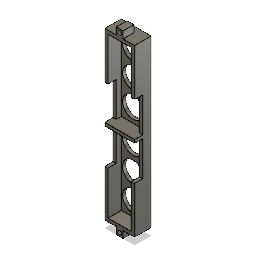
_Tamed Tiger.d4603d96-84c6-47e9-a002-08c8963379fb (Autodesk Fusion 360 design; units mm, degrees)
Autodesk Fusion 360 part; units mm, degrees
sketch "Sketch1" plane through (0, 0, 0) normal (0, 0, 1) x (1, 0, 0) in component "Chassis"
  line L0 (0, 0) -> (142, 0)
  line L1 (142, 0) -> (142, 170)
  line L2 (142, 170) -> (0, 170)
  line L3 (0, 170) -> (0, 0)
  line L4 (3, 3) -> (139, 3)
  line L5 (139, 3) -> (139, 167)
  line L6 (139, 167) -> (3, 167)
  line L7 (3, 167) -> (3, 3)
  line L8 (35, 154) -> (55, 154)
  line L9 (58, 86.5) -> (32, 86.5)
  line L10 (35, 86.5) -> (35, 142)
  line L11 (32, 142) -> (32, 167)
  line L12 (32, 157) -> (58, 157)
  line L13 (58, 167) -> (58, 85)
  line L14 (32, 85) -> (32, 142)
  line L15 (58, 3) -> (58, 85)
  line L16 (35, 83.5) -> (35, 28)
  line L17 (32, 28) -> (32, 3)
  line L18 (32, 13) -> (58, 13)
  line L19 (35, 16) -> (55, 16)
  line L20 (32, 85) -> (32, 28)
  line L21 (35, 142) -> (35, 154)
  line L22 (35, 157) -> (35, 167)
  line L23 (55, 167) -> (55, 157)
  line L24 (55, 154) -> (55, 86.5)
  line L25 (35, 28) -> (35, 16)
  line L26 (35, 13) -> (35, 3)
  line L27 (55, 3) -> (55, 13)
  line L28 (55, 16) -> (55, 83.5)
  line L29 (84, 86.5) -> (110, 86.5)
  line L30 (87, 154) -> (87, 86.5)
  line L31 (107, 86.5) -> (107, 142)
  line L32 (84, 167) -> (84, 85)
  line L33 (110, 28) -> (110, 3)
  line L34 (107, 157) -> (107, 167)
  line L35 (107, 16) -> (87, 16)
  line L36 (110, 85) -> (110, 142)
  line L37 (110, 157) -> (84, 157)
  line L38 (87, 167) -> (87, 157)
  line L39 (110, 13) -> (84, 13)
  line L40 (87, 3) -> (87, 13)
  line L41 (107, 28) -> (107, 16)
  line L42 (107, 142) -> (107, 154)
  line L43 (87, 16) -> (87, 83.5)
  line L44 (107, 83.5) -> (107, 28)
  line L45 (110, 85) -> (110, 28)
  line L46 (107, 154) -> (87, 154)
  line L47 (107, 13) -> (107, 3)
  line L48 (110, 142) -> (110, 167)
  line L49 (84, 3) -> (84, 85)
  line L50 (45, 163) -> (48, 163)
  line L51 (48, 163) -> (42, 163)
  line L52 (42, 163) -> (42, 157)
  line L53 (42, 157) -> (48, 157)
  line L54 (48, 157) -> (48, 163)
  line L55 (97, 163) -> (100, 163)
  line L56 (100, 163) -> (94, 163)
  line L57 (94, 163) -> (94, 157)
  line L58 (94, 157) -> (100, 157)
  line L59 (100, 157) -> (100, 163)
  line L60 (97, 7) -> (100, 7)
  line L61 (45, 7) -> (48, 7)
  line L62 (48, 7) -> (42, 7)
  line L63 (42, 7) -> (42, 13)
  line L64 (42, 13) -> (48, 13)
  line L65 (48, 13) -> (48, 7)
  line L66 (100, 7) -> (94, 7)
  line L67 (94, 7) -> (94, 13)
  line L68 (94, 13) -> (100, 13)
  line L69 (100, 13) -> (100, 7)
  line L70 (110, 83.5) -> (84, 83.5)
  line L71 (58, 83.5) -> (32, 83.5)
  line L72 (58, 53.5) -> (55, 53.5)
  line L73 (35, 53.5) -> (32, 53.5)
  line L74 (58, 116.5) -> (55, 116.5)
  line L75 (35, 116.5) -> (32, 116.5)
  line L76 (84, 116.5) -> (87, 116.5)
  line L77 (107, 116.5) -> (110, 116.5)
  line L78 (110, 53.5) -> (107, 53.5)
  line L79 (87, 53.5) -> (84, 53.5)
  line L80 (84, 3) -> (58, 3)
  line L81 (58, 3) -> (58, 6)
  line L82 (58, 6) -> (84, 6)
  line L83 (84, 6) -> (84, 3)
  line L84 (84, 167) -> (58, 167)
  line L85 (58, 167) -> (58, 164)
  line L86 (58, 164) -> (84, 164)
  line L87 (84, 164) -> (84, 167)
  line L88 (136, 80) -> (139, 80)
  line L89 (136, 90) -> (139, 90)
  line L90 (139, 90) -> (136, 90)
  line L91 (136, 90) -> (136, 80)
  line L92 (136, 80) -> (139, 80)
  line L93 (139, 80) -> (139, 90)
  line L94 (6, 85) -> (6, 90)
  line L95 (6, 90) -> (3, 90)
  line L96 (3, 90) -> (3, 80)
  line L97 (3, 80) -> (6, 80)
  line L98 (6, 80) -> (6, 90)
  line L99 (84, 90) -> (81, 90)
  line L100 (81, 90) -> (84, 90)
  line L101 (81, 80) -> (84, 80)
  line L102 (81, 80) -> (84, 80)
  line L103 (84, 80) -> (84, 90)
  line L104 (58, 90) -> (58, 80)
  line L105 (58, 80) -> (61, 80)
  line L106 (61, 90) -> (58, 90)
  line L107 (78, 90) -> (81, 90)
  line L108 (78, 80) -> (81, 80)
  line L109 (81, 90) -> (78, 90)
  line L110 (78, 90) -> (78, 80)
  line L111 (78, 80) -> (81, 80)
  line L112 (64, 80) -> (64, 90)
  line L113 (61, 80) -> (64, 80)
  line L114 (64, 85) -> (64, 90)
  line L115 (64, 90) -> (61, 90)
  circle A0 centre (81, 85) radius 1.6
  circle A1 centre (61, 85) radius 1.6
  dimension "d1" = 170
  dimension "d2" = 142
  dimension "d12" = -3
  dimension "d13" = 12
  dimension "d14" = 20
  dimension "d15" = 67.5
  dimension "d16" = 20
  dimension "d46" = 3
  dimension "d47" = 6
  dimension "d49" = 3
  dimension "d50" = 6
  dimension "d53" = 3
  dimension "d54" = 6
  dimension "d55" = 6
  dimension "d250" = 3
  dimension "d251" = 3
  dimension "d254" = 3
  dimension "d256" = 5
  dimension "d257" = 10
  dimension "d262" = 3
  dimension "d264" = 10
  dimension "d265" = 3
  dimension "d267" = 10
  dimension "d295" = 3.2
  dimension "d296" = 3.2
  constraint horizontal L0
  constraint vertical L1
  constraint horizontal L2
  constraint vertical L3
  constraint coincident L0.start L3.end
  constraint perpendicular L8 L21
  constraint perpendicular L8 L23
  constraint perpendicular L9 L23
  constraint parallel L11 L21
  constraint parallel L8 L12
  constraint parallel L13 L23
  constraint parallel L10 L14
  constraint coincident L12.start L11
  constraint coincident L6 L11.end
  constraint coincident L6 L22.end
  constraint coincident L18.start L17
  constraint coincident L4 L17.end
  constraint coincident L4 L26.end
  constraint coincident L19.end L27
  constraint coincident L4 L27.start
  constraint coincident L18.end L15
  constraint coincident L4 L15.start
  constraint coincident L12.end L13
  constraint coincident L6 L13.start
  constraint coincident L8.end L23
  constraint coincident L6 L23.start
  constraint coincident L12 L22.start
  constraint collinear L21 L22
  constraint coincident L12 L23.end
  constraint collinear L23 L24
  constraint coincident L18 L26.start
  constraint collinear L25 L26
  constraint coincident L18 L27.end
  constraint collinear L27 L28
  constraint horizontal L51
  constraint vertical L52
  constraint horizontal L53
  constraint vertical L54
  constraint horizontal L56
  constraint vertical L57
  constraint horizontal L58
  constraint vertical L59
  constraint horizontal L62
  constraint vertical L63
  constraint horizontal L64
  constraint vertical L65
  constraint horizontal L66
  constraint vertical L67
  constraint horizontal L68
  constraint vertical L69
  constraint coincident L28.end L70
  constraint coincident L16.start L70
  constraint coincident L10.start L9
  constraint coincident L13 L9.start
  constraint coincident L24.end L9
  constraint coincident L32 L29.start
  constraint coincident L30.end L29
  constraint coincident L44.start L70
  constraint coincident L31.start L29
  constraint coincident L49 L70.end
  constraint coincident L15 L71.start
  constraint collinear L70 L71
  constraint parallel L71 L72
  constraint coincident L28 L72.end
  constraint coincident L16 L73.start
  constraint collinear L72 L73
  constraint parallel L9 L74
  constraint coincident L24 L74.end
  constraint coincident L10 L75.start
  constraint collinear L74 L75
  constraint parallel L29 L76
  constraint coincident L30 L76.end
  constraint coincident L31 L77.start
  constraint collinear L76 L77
  constraint parallel L70 L78
  constraint coincident L44 L78.end
  constraint coincident L43 L79.start
  constraint collinear L78 L79
  constraint horizontal L80
  constraint vertical L81
  constraint horizontal L82
  constraint vertical L83
  constraint horizontal L84
  constraint vertical L85
  constraint horizontal L86
  constraint vertical L87
  constraint horizontal L90
  constraint vertical L91
  constraint horizontal L92
  constraint vertical L93
  constraint horizontal L95
  constraint vertical L96
  constraint horizontal L97
  constraint vertical L98
  constraint horizontal L99
  constraint horizontal L101
  constraint vertical L103
  constraint horizontal L106
  constraint vertical L104
  constraint horizontal L105
  constraint horizontal L109
  constraint vertical L110
  constraint horizontal L111
  constraint horizontal L115
  constraint horizontal L113
  constraint vertical L112
  measures "d1" distance of L0.start L2.end
  measures "d2" distance of L0.start L0.end
  measures "d13" distance of L10.end L8.start
  measures "d14" distance of L8.start L8.end
  measures "d15" distance of L8.end L24.end
  measures "d16" distance of L24.end L10.start
  measures "d46" distance of L50.start L50.end
  measures "d47" distance of L50.end L51.end
  measures "d49" distance of L55.start L55.end
  measures "d50" distance of L55.end L56.end
  measures "d53" distance of L61.start L61.end
  measures "d54" distance of L61.end L62.end
  measures "d55" distance of L60.end L66.end
  measures "d250" distance of L49.start L82.end
  measures "d251" distance of L32.start L86.end
  measures "d254" distance of L89.end L89.start
  measures "d256" distance of L94.start L94.end
  measures "d257" distance of L94.end L97.end
  measures "d262" distance of L99.end L99.start
  measures "d264" distance of L105.end L106.start
  measures "d265" distance of L107.start L99.end
  measures "d267" distance of L112.start L112.end
  measures "d295" diameter of A0
  measures "d296" diameter of A1
extrude "Extrude4" add sketch "Sketch1" along normal blind 3 contours L16 L19 L25 L28 L71 | L8 L9 L10 L21 L24 | L35 L41 L43 L44 L70 | L29 L30 L31 L42 L46 makes body 1 at (100.3333, 109, 0) makes body 2 at (100.3333, 61, 0) makes body 3 at (41.6667, 109, 0) makes body 4 at (41.6667, 61, 0) in component "Chassis"
extrude "Extrude1" add sketch "Sketch1" along normal blind 39 separate body contours L0 L1 L2 L3 makes body 5 in component "Chassis"
sketch "Sketch2" plane through (0, 0, 0) normal (1, 0, 0) x (0, 0, -1) in component "Chassis"
  line L0 (17, 142) -> (21.5, 142)
  line L1 (33, 154) -> (33, 86.5)
  line L2 (33, 86.5) -> (10, 86.5)
  line L3 (10, 86.5) -> (10, 154)
  line L4 (33, 154) -> (10, 154)
  line L5 (10, 16) -> (10, 83.5)
  line L6 (10, 83.5) -> (33, 83.5)
  line L7 (33, 83.5) -> (33, 16)
  line L8 (33, 16) -> (10, 16)
  line L9 (21.5, 3) -> (21.5, 167)
  circle A0 centre (21.5, 28) radius 4.5
  circle A1 centre (21.5, 142) radius 4.5
  line L10 (0, 170) -> (0, 0)
  line L11 (2, 170) -> (41, 170)
  line L12 (2, 0) -> (41, 0)
  line L13 (41, 0) -> (41, 170)
  line L14 (2, 0) -> (2, 170)
  line L15 (5, 167) -> (38, 167)
  line L16 (38, 3) -> (38, 167)
  line L17 (5, 3) -> (38, 3)
  line L18 (5, 3) -> (5, 167)
  line L19 (7, 86.5) -> (7, 157)
  line L20 (36, 157) -> (7, 157)
  line L21 (36, 157) -> (36, 86.5)
  line L22 (36, 83.5) -> (36, 13)
  line L23 (36, 13) -> (7, 13)
  arc A2 (2, 129.8037) -> (5, 125.9766) centre (21.5, 142) ccw
  arc A3 (38, 125.9766) -> (41, 129.8037) centre (21.5, 142) ccw
  arc A4 (41, 154.1963) -> (38, 158.0234) centre (21.5, 142) ccw
  arc A5 (5, 158.0234) -> (2, 154.1963) centre (21.5, 142) ccw
  arc A6 (38, 11.9766) -> (41, 15.8037) centre (21.5, 28) ccw
  arc A7 (2, 15.8037) -> (5, 11.9766) centre (21.5, 28) ccw
  arc A8 (41, 40.1963) -> (38, 44.0234) centre (21.5, 28) ccw
  arc A9 (5, 44.0234) -> (2, 40.1963) centre (21.5, 28) ccw
  line L24 (17, 28) -> (21.5, 28)
  line L25 (7, 13) -> (7, 83.5)
  line L26 (36, 86.5) -> (36, 83.5)
  line L27 (7, 86.5) -> (7, 83.5)
  point P0 (0, 142)
  point P1 (0, 28)
  point P2 (0, 170)
  dimension "d18" = 21.5
  dimension "d21" = 67.5
  dimension "d22" = 23
  dimension "d23" = 67.5
  dimension "d26" = 67.5
  dimension "d27" = 23
  dimension "d28" = 67.5
  dimension "d29" = 9
  dimension "d30" = 9
  dimension "d35" = -3
  dimension "d36" = -3
  dimension "d40" = 70.5
  constraint perpendicular L1 L2
  constraint perpendicular L2 L3
  constraint perpendicular L5 L6
  constraint perpendicular L6 L7
  constraint perpendicular L4 L9
  constraint coincident A0.centre A6.centre
  constraint perpendicular L10 L11
  constraint perpendicular L10 L12
  constraint parallel L7 L22
  constraint parallel L8 L23
  constraint coincident L17 L9.start
  constraint coincident L15 L9.end
  constraint coincident L13 A3.end
  constraint coincident L13 A4.start
  constraint concentric A2 A4
  constraint coincident L14 A2.start
  constraint coincident L14 A5.end
  constraint coincident L18 A2.end
  constraint concentric A2 A3
  constraint coincident L16 A3.start
  constraint coincident L16 A4.end
  constraint concentric A4 A5
  constraint coincident L18 A5.start
  constraint coincident L18 A7.end
  constraint coincident L16 A6.start
  constraint coincident L13 A6.end
  constraint coincident L13 A8.start
  constraint concentric A6 A8
  constraint concentric A7 A8
  constraint coincident L14 A9.end
  constraint coincident L14 A7.start
  constraint coincident L18 A9.start
  constraint concentric A8 A9
  constraint coincident A1 L0.start
  constraint coincident A0 L24.start
  constraint coincident L16 A8.end
  constraint perpendicular L23 L25
  constraint parallel L22 L26
  constraint parallel L25 L27
  measures "d18" distance of P1 A0.centre
  measures "d21" distance of L1.start L1.end
  measures "d22" distance of L1.end L2.end
  measures "d23" distance of L2.end L3.end
  measures "d26" distance of L5.start L5.end
  measures "d27" distance of L5.end L6.end
  measures "d28" distance of L6.end L7.end
  measures "d29" diameter of A0
  measures "d30" diameter of A1
  measures "d40" distance of L23.end L25.end
extrude "Extrude2" add sketch "Sketch1" along normal blind 3 contours L4 L6 L7 L11 L14 L17 L20 L94 L95 L97 L98 | L7 L94 L95 L96 L97 L98 | L4 L18 L26 L27 L61 L62 L63 L65 | L4 L15 L49 L80 L81 L82 L83 | L18 L61 L62 L63 L64 L65 | L13 L15 L32 L49 L82 L86 L99 L100 L101 L102 L105 L106 L107 L108 L109 L110 L111 L112 L113 L114 L115 | L6 L12 L22 L23 L50 L51 L52 L54 | L4 L39 L40 L47 L60 L66 L67 L69 | L13 L15 L104 L105 L106 L112 L113 L114 L115 | L6 L13 L32 L84 L85 L86 L87 | L12 L50 L51 L52 L53 L54 | L4 L5 L6 L33 L36 L45 L48 L88 L89 L90 L91 L92 | L39 L60 L66 L67 L68 L69 | L32 L49 L99 L100 L101 L102 L103 L107 L108 L109 L110 L111 | L6 L34 L37 L38 L55 L56 L57 L59 | L5 L88 L89 L90 L91 L92 L93 | L37 L55 L56 L57 L58 L59 | A0 | A1 bodies 5 in component "Chassis"
extrude "Extrude1'" add sketch "Sketch1" along normal blind 3 separate body contours L16 L19 L25 L28 L71 | L8 L9 L10 L21 L24 | L35 L41 L43 L44 L70 | L29 L30 L31 L42 L46 makes body 6 at (100.3333, 61, 0) makes body 7 at (41.6667, 61, 0) makes body 8 at (100.3333, 109, 0) makes body 9 at (41.6667, 109, 0)
extrude "Extrude3" add sketch "Sketch1" along normal blind 19.5 contours L4 L17 L18 L26 | L15 L16 L17 L18 L19 L20 L25 L28 L64 L72 L73 | L4 L15 L18 L27 L81 | L16 L20 L71 L73 | L6 L11 L12 L22 | L4 L39 L40 L49 L83 | L9 L13 L14 L15 L20 L71 L104 | L8 L10 L11 L12 L13 L14 L21 L24 L53 L74 L75 | L15 L28 L71 L72 L104 | L6 L12 L13 L23 L85 | L4 L33 L39 L47 | L33 L35 L39 L41 L43 L44 L45 L49 L68 L78 L79 | L9 L10 L14 L75 | L43 L49 L70 L79 L103 | L6 L32 L37 L38 L87 | L35 L41 L43 L44 L70 | L9 L13 L24 L74 L104 | L29 L32 L36 L45 L49 L70 L103 | L6 L34 L37 L48 | L30 L31 L32 L36 L37 L42 L46 L48 L58 L76 L77 | L44 L45 L70 L78 | L29 L30 L32 L76 L103 | L29 L31 L36 L77 bodies 5 in component "Chassis"
copy_body "CutPasteBodies1" bodies 6 5 7 8 9 removing the originals makes body 10 makes body 11 makes body 12 makes body 13 makes body 14 in component "Chassis"
combine "Combine1" operation add target body 10 tool bodies 13 14 11 12 in component "Chassis"
extrude "Extrude5" add sketch "Sketch1" along normal blind 10 separate body contours L18 L61 L62 L63 L64 L65 | L12 L50 L51 L52 L53 L54 | L39 L60 L66 L67 L68 L69 | L37 L55 L56 L57 L58 L59 makes body 15 at (94, 161, 3.3333) makes body 16 at (98, 13, 3.3333) makes body 17 at (42, 161, 3.3333) makes body 18 at (44, 13, 3.3333) in component "Chassis"
move_body "Move1" bodies 18 16 17 15 to x (1, 0, 0) y (0, 1, 0) z (0, 0, 1) at (0, 0, 9.5) in component "Chassis"
move_body "Move2" bodies 4 3 2 1 to x (1, 0, 0) y (0, 1, 0) z (0, 0, 1) at (0, 0, 5.5) in component "Chassis"
move_body "Move3" bodies 1 2 3 4 to x (1, 0, 0) y (0, 1, 0) z (0, 0, 1) at (0, 0, -0.5) in component "Chassis"
combine "Combine2" operation add target body 1 tool bodies 17 15 16 10 18 2 3 4 in component "Chassis"
hole "Hole1" at (45, 142, 8) direction (0, 0, -1) diameter 18 depth 3 tip angle 180 bodies 1 in component "Chassis"
hole "Hole2" at (45, 98.5, 8) direction (0, 0, -1) diameter 18 depth 3 tip angle 180 bodies 1 in component "Chassis"
hole "Hole3" at (45, 120, 8) direction (0, 0, -1) diameter 18 depth 3 tip angle 180 bodies 1 in component "Chassis"
hole "Hole4" at (97, 142, 8) direction (0, 0, -1) diameter 18 depth 3 tip angle 180 bodies 1 in component "Chassis"
hole "Hole5" at (97, 98.5, 8) direction (0, 0, -1) diameter 18 depth 3 tip angle 180 bodies 1 in component "Chassis"
hole "Hole6" at (97, 120.5, 8) direction (0, 0, -1) diameter 18 depth 3 tip angle 180 bodies 1 in component "Chassis"
hole "Hole7" at (45, 71.5, 8) direction (0, 0, -1) diameter 18 depth 3 tip angle 180 bodies 1 in component "Chassis"
hole "Hole8" at (45, 71.5, 8) direction (0, 0, -1) diameter 18 depth 3 tip angle 180 bodies 1 in component "Chassis"
hole "Hole9" at (45, 49.5, 8) direction (0, 0, -1) diameter 18 depth 3 tip angle 180 bodies 1 in component "Chassis"
hole "Hole10" at (45, 28, 8) direction (0, 0, -1) diameter 18 depth 3 tip angle 180 bodies 1 in component "Chassis"
hole "Hole12" at (45, 28, 8) direction (0, 0, -1) diameter 18 depth 3 tip angle 180 bodies 1 in component "Chassis"
hole "Hole17" at (45, 160, 19.5) direction (0, 0, -1) diameter 2.9 depth 12 tip angle 180 bodies 1 in component "Chassis"
hole "Hole18" at (97, 160, 19.5) direction (0, 0, -1) diameter 2.9 depth 12 tip angle 180 bodies 1 in component "Chassis"
hole "Hole19" at (97, 10, 19.5) direction (0, 0, -1) diameter 2.9 depth 12 tip angle 180 bodies 1 in component "Chassis"
hole "Hole20" at (45, 10, 19.5) direction (0, 0, -1) diameter 2.9 depth 12 tip angle 180 bodies 1 in component "Chassis"
extrude "Extrude6" cut sketch "Sketch1" along normal blind 30 contours L16 L20 L71 L73 | L16 L19 L25 L28 L71 | L15 L28 L71 L72 L104 | L9 L10 L14 L75 | L43 L49 L70 L79 L103 | L9 L13 L24 L74 L104 | L44 L45 L70 L78 | L29 L30 L32 L76 L103 | L29 L31 L36 L77 bodies 1 in component "Chassis"
extrude "Extrude7" add sketch "Sketch1" along normal blind 3 contours L16 L19 L25 L28 L71 bodies 1 in component "Chassis"
extrude "Extrude8" cut sketch "Sketch1" along normal blind 30 contours L35 L41 L43 L44 L70 bodies 1 in component "Chassis"
extrude "Extrude9" add sketch "Sketch1" along normal blind 3 contours L35 L41 L43 L44 L70 bodies 1 in component "Chassis"
extrude "Extrude10" add sketch "Sketch1" along normal blind 12.5 contours L16 L20 L71 L73 | L15 L28 L71 L72 L104 | L9 L10 L14 L75 | L43 L49 L70 L79 L103 | L9 L13 L24 L74 L104 | L44 L45 L70 L78 | L29 L30 L32 L76 L103 | L29 L31 L36 L77 bodies 1 in component "Chassis"
extrude "Extrude11" add sketch "Sketch1" along normal blind 8 contours L16 L19 L25 L28 L71 | L35 L41 L43 L44 L70 bodies 1 in component "Chassis"
extrude "Extrude12" cut sketch "Sketch1" along normal blind 5 contours L16 L19 L25 L28 L71 | L35 L41 L43 L44 L70 bodies 1 in component "Chassis"
extrude "Extrude13" add sketch "Sketch1" along normal blind 3 contours L16 L19 L25 L28 L71 | L35 L41 L43 L44 L70 bodies 1 in component "Chassis"
hole "Hole21" at (45, 28, 8) direction (0, 0, -1) diameter 18 depth 3 tip angle 180 bodies 1 in component "Chassis"
hole "Hole22" at (45, 50, 8) direction (0, 0, -1) diameter 18 depth 3 tip angle 180 bodies 1 in component "Chassis"
hole "Hole23" at (45, 71.5, 8) direction (0, 0, -1) diameter 18 depth 3 tip angle 180 bodies 1 in component "Chassis"
hole "Hole24" at (97, 28, 8) direction (0, 0, -1) diameter 18 depth 3 tip angle 180 bodies 1 in component "Chassis"
hole "Hole25" at (97, 50, 8) direction (0, 0, -1) diameter 18 depth 3 tip angle 180 bodies 1 in component "Chassis"
hole "Hole26" at (97, 71.5, 8) direction (0, 0, -1) diameter 18 depth 3 tip angle 180 bodies 1 in component "Chassis"
extrude "Extrude2'" add sketch "Sketch1" along normal blind 39 separate body contours L4 L6 L7 L11 L14 L17 L20 L94 L95 L97 L98 | L4 L17 L18 L26 | L7 L94 L95 L96 L97 L98 | L4 L18 L26 L27 L61 L62 L63 L65 | L15 L16 L17 L18 L19 L20 L25 L28 L64 L72 L73 | L4 L15 L18 L27 L81 | L4 L15 L49 L80 L81 L82 L83 | L18 L61 L62 L63 L64 L65 | L16 L20 L71 L73 | L6 L11 L12 L22 | L4 L39 L40 L49 L83 | L13 L15 L32 L49 L82 L86 L99 L100 L101 L102 L105 L106 L107 L108 L109 L110 L111 L112 L113 L114 L115 | L9 L13 L14 L15 L20 L71 L104 | L16 L19 L25 L28 L71 | L6 L12 L22 L23 L50 L51 L52 L54 | L8 L10 L11 L12 L13 L14 L21 L24 L53 L74 L75 | L4 L39 L40 L47 L60 L66 L67 L69 | L15 L28 L71 L72 L104 | L6 L12 L13 L23 L85 | L4 L33 L39 L47 | L33 L35 L39 L41 L43 L44 L45 L49 L68 L78 L79 | L13 L15 L104 L105 L106 L112 L113 L114 L115 | L9 L10 L14 L75 | L6 L13 L32 L84 L85 L86 L87 | L12 L50 L51 L52 L53 L54 | L4 L5 L6 L33 L36 L45 L48 L88 L89 L90 L91 L92 | L39 L60 L66 L67 L68 L69 | L43 L49 L70 L79 L103 | L8 L9 L10 L21 L24 | L6 L32 L37 L38 L87 | L32 L49 L99 L100 L101 L102 L103 L107 L108 L109 L110 L111 | L35 L41 L43 L44 L70 | L9 L13 L24 L74 L104 | L6 L34 L37 L38 L55 L56 L57 L59 | L5 L88 L89 L90 L91 L92 L93 | L29 L32 L36 L45 L49 L70 L103 | L6 L34 L37 L48 | L30 L31 L32 L36 L37 L42 L46 L48 L58 L76 L77 | L44 L45 L70 L78 | L37 L55 L56 L57 L58 L59 | L29 L30 L32 L76 L103 | L29 L30 L31 L42 L46 | L29 L31 L36 L77 | A0 | A1 makes body 19
extrude "Extrude3'" cut sketch "Sketch1" along normal blind 36 contours L4 L6 L7 L11 L14 L17 L20 L94 L95 L97 L98 | L4 L17 L18 L26 | L7 L94 L95 L96 L97 L98 | L4 L18 L26 L27 L61 L62 L63 L65 | L15 L16 L17 L18 L19 L20 L25 L28 L64 L72 L73 | L4 L15 L18 L27 L81 | L4 L15 L49 L80 L81 L82 L83 | L18 L61 L62 L63 L64 L65 | L16 L20 L71 L73 | L6 L11 L12 L22 | L4 L39 L40 L49 L83 | L13 L15 L32 L49 L82 L86 L99 L100 L101 L102 L105 L106 L107 L108 L109 L110 L111 L112 L113 L114 L115 | L9 L13 L14 L15 L20 L71 L104 | L16 L19 L25 L28 L71 | L6 L12 L22 L23 L50 L51 L52 L54 | L8 L10 L11 L12 L13 L14 L21 L24 L53 L74 L75 | L4 L39 L40 L47 L60 L66 L67 L69 | L15 L28 L71 L72 L104 | L6 L12 L13 L23 L85 | L4 L33 L39 L47 | L33 L35 L39 L41 L43 L44 L45 L49 L68 L78 L79 | L13 L15 L104 L105 L106 L112 L113 L114 L115 | L9 L10 L14 L75 | L6 L13 L32 L84 L85 L86 L87 | L12 L50 L51 L52 L53 L54 | L4 L5 L6 L33 L36 L45 L48 L88 L89 L90 L91 L92 | L39 L60 L66 L67 L68 L69 | L43 L49 L70 L79 L103 | L8 L9 L10 L21 L24 | L6 L32 L37 L38 L87 | L32 L49 L99 L100 L101 L102 L103 L107 L108 L109 L110 L111 | L35 L41 L43 L44 L70 | L9 L13 L24 L74 L104 | L6 L34 L37 L38 L55 L56 L57 L59 | L5 L88 L89 L90 L91 L92 L93 | L29 L32 L36 L45 L49 L70 L103 | L6 L34 L37 L48 | L30 L31 L32 L36 L37 L42 L46 L48 L58 L76 L77 | L44 L45 L70 L78 | L37 L55 L56 L57 L58 L59 | L29 L30 L32 L76 L103 | L29 L30 L31 L42 L46 | L29 L31 L36 L77 | A0 | A1 bodies 19
copy_body "Body->Comp1" bodies 19 removing the originals makes body 20 in component "lid"
hole "Hole27" at (107, 28, 19.5) direction (1, 0, 0) diameter 45 depth 27 tip angle 180 bodies 1 in component "Chassis"
hole "Hole1'" at (107, 28, 19.5) direction (1, 0, 0) diameter 45 depth 27 tip angle 180 bodies 20 in component "lid"
hole "Hole28" at (35, 28, 19.5) direction (-1, 0, 0) diameter 45 depth 27 tip angle 180 bodies 1 in component "Chassis"
hole "Hole2'" at (35, 28, 19.5) direction (-1, 0, 0) diameter 45 depth 27 tip angle 180 bodies 20 in component "lid"
hole "Hole29" at (35, 142, 19.5) direction (-1, 0, 0) diameter 45 depth 27 tip angle 180 bodies 1 in component "Chassis"
hole "Hole3'" at (35, 142, 19.5) direction (-1, 0, 0) diameter 45 depth 27 tip angle 180 bodies 20 in component "lid"
hole "Hole30" at (107, 142, 19.5) direction (1, 0, 0) diameter 45 depth 27 tip angle 180 bodies 1 in component "Chassis"
hole "Hole4'" at (107, 142, 19.5) direction (1, 0, 0) diameter 45 depth 27 tip angle 180 bodies 20 in component "lid"
extrude "Extrude14" add sketch "Sketch1" along normal blind 19.5 contours L15 L16 L17 L18 L19 L20 L25 L28 L64 L72 L73 | L8 L10 L11 L12 L13 L14 L21 L24 L53 L74 L75 | L33 L35 L39 L41 L43 L44 L45 L49 L68 L78 L79 | L30 L31 L32 L36 L37 L42 L46 L48 L58 L76 L77 bodies 1 in component "Chassis"
extrude "Extrude15" add sketch "Sketch1" along normal blind 19.5 contours L4 L17 L18 L26 | L6 L11 L12 L22 | L4 L33 L39 L47 | L6 L34 L37 L48 bodies 1 in component "Chassis"
extrude "Extrude16" cut sketch "Sketch1" along normal blind 36 contours L7 L94 L95 L96 L97 L98 | L4 L15 L49 L80 L81 L82 L83 | L6 L13 L32 L84 L85 L86 L87 | L5 L88 L89 L90 L91 L92 L93 bodies 1 in component "Chassis"
extrude "Extrude17" add sketch "Sketch1" along normal blind 36 contours L7 L94 L95 L96 L97 L98 | L4 L15 L49 L80 L81 L82 L83 | L6 L13 L32 L84 L85 L86 L87 | L5 L88 L89 L90 L91 L92 L93 bodies 1 in component "Chassis"
extrude "Extrude18" add sketch "Sketch1" along normal blind 36 contours L13 L15 L104 L105 L106 L112 L113 L114 L115 | L32 L49 L99 L100 L101 L102 L103 L107 L108 L109 L110 L111 | A0 | A1 bodies 1 in component "Chassis"
hole "Hole31" at (32, 28, 19.5) direction (1, 0, 0) diameter 9 depth 78 tip angle 180 bodies 1 in component "Chassis"
hole "Hole32" at (110, 142, 19.5) direction (-1, 0, 0) diameter 9 depth 78 tip angle 180 bodies 1 in component "Chassis"
hole "Hole33" at (0, 142, 19.5) direction (1, 0, 0) diameter 3 depth 150 tip angle 180 bodies 1 in component "Chassis"
hole "Hole34" at (0, 28, 19.5) direction (1, 0, 0) diameter 3 depth 150 tip angle 180 bodies 1 in component "Chassis"
hole "Hole35" at (61, 85, 36) direction (0, 0, -1) diameter 3 depth 20 tip angle 180 bodies 1 in component "Chassis"
hole "Hole36" at (81, 85, 36) direction (0, 0, -1) diameter 3 depth 20 tip angle 180 bodies 1 in component "Chassis"
extrude "Extrude1''" cut sketch "Sketch1" along normal blind 40 contours A0 | A1 bodies 20 in component "lid"
extrude "Extrude9'" add sketch "Sketch1" along normal blind 14.5 separate body contours L15 L16 L17 L18 L19 L20 L25 L28 L64 L72 L73 | L18 L61 L62 L63 L64 L65 | L9 L13 L14 L15 L20 L71 L104 | L8 L10 L11 L12 L13 L14 L21 L24 L53 L74 L75 | L12 L50 L51 L52 L53 L54 makes body 21 at (32, 40, 4.8333) makes body 22 at (49.3333, 86.5, 9.6667) makes body 23 at (32, 130, 4.8333)
extrude "Extrude10'" add sketch "Sketch1" along normal blind 7.5 contours L16 L20 L71 L73 | L15 L28 L71 L72 L104 | L9 L10 L14 L75 | L9 L13 L24 L74 L104 bodies 21 22 23
extrude "Extrude11'" add sketch "Sketch1" along normal blind 3 contours L16 L19 L25 L28 L71 | L8 L9 L10 L21 L24 bodies 21
extrude "Extrude12'" cut sketch "Sketch1" along normal blind 5 contours L18 L61 L62 L63 L64 L65 | L12 L50 L51 L52 L53 L54 bodies 21
copy_body "Body->Comp3" bodies 21 removing the originals makes body 24 in component "motor cover"
hole "Hole1''" at (45, 28, 3) direction (0, 0, -1) diameter 18 depth 20 tip angle 180 bodies 24 in component "motor cover"
hole "Hole2''" at (45, 49.75, 3) direction (0, 0, -1) diameter 18 depth 20 tip angle 180 bodies 24 in component "motor cover"
hole "Hole3''" at (45, 71.5, 3) direction (0, 0, -1) diameter 18 depth 20 tip angle 180 bodies 24 in component "motor cover"
hole "Hole4''" at (45, 142, 3) direction (0, 0, -1) diameter 18 depth 20 tip angle 180 bodies 24 in component "motor cover"
hole "Hole5'" at (45, 120.25, 3) direction (0, 0, -1) diameter 18 depth 20 tip angle 180 bodies 24 in component "motor cover"
hole "Hole6'" at (45, 98.5, 3) direction (0, 0, -1) diameter 18 depth 20 tip angle 180 bodies 24 in component "motor cover"
hole "Hole7'" at (45, 160, 14.5) direction (0, 0, -1) diameter 3.2 depth 20 tip angle 180 bodies 24 in component "motor cover"
hole "Hole8'" at (45, 10, 14.5) direction (0, 0, -1) diameter 3.2 depth 20 tip angle 180 bodies 24 in component "motor cover"
component "Chassis" placed x (1, 0, 0) y (0, 1, 0) z (0, 0, 1) at (0, 0, 0)
component "lid" placed x (1, 0, 0) y (0, 1, 0) z (0, 0, 1) at (0, 0, 0)
component "motor cover" placed x (1, 0, 0) y (0, 1, 0) z (0, 0, 1) at (0, 0, 0)
named bodies: "lid"
